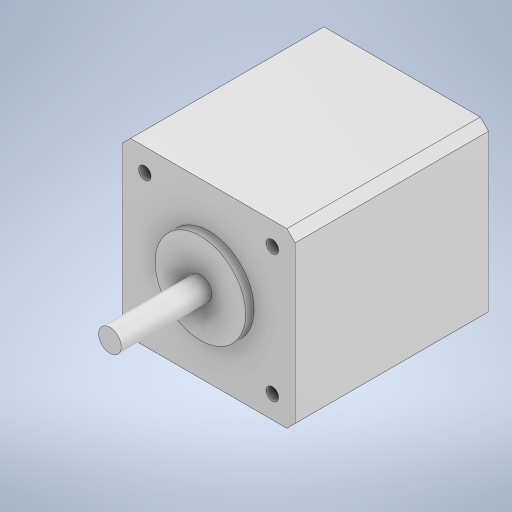
# Autodesk Inventor part: stepper motor
Saved by Autodesk Inventor 2024 (Build 280153000, 153)
## iProperties
Created: 2023-10-25
Part Number: stepper motor
Material: Aluminum
Document SubType Name: Modeling
Designer: mb
Density: 2.7 g/cm^3
Appearance: Satin
Mass: 225.957 g
Surface Area: 118.758 cm^2
Volume: 83.6877 cm^3
Author: mb
Autodesk Inventor part; units mm, degrees
ref_plane "YZ Plane" through (0, 0, 0) normal (1, 0, 0) x (0, 1, 0)
sketch "Sketch1" plane through (0, 0, 0) normal (0, 0, 1) x (1, 0, 0)
  line L0 (0, 0) -> (42, 0)
  line L1 (42, 0) -> (42, 42)
  line L2 (42, 42) -> (0, 42)
  line L3 (0, 42) -> (0, 0)
  dimension "d0" = 42
  dimension "d1" = 42
  constraints: 8 end point, 2 parallel, 1 horizontal, 1 perpendicular
  measures "d0" distance of L2.end L1.end
  measures "d1" distance of L1.end L0.end
extrude "Extrusion1" add sketch "Sketch1" along normal blind 47
chamfer "Chamfer1" distance 2 angle 45 4 edges at (42, 42, 23.5) (0, 42, 23.5) (42, 0, 23.5) (0, 0, 23.5)
sketch "Sketch2" plane through (0, 0, 47) normal (0, 0, 1) x (1, 0, 0)
  circle A0 centre (21, 21) radius 11
  line L0 (42, 2) -> (42, 40) projected
  line L1 (40, 42) -> (2, 42) projected
  point P0 (0, 0)
  point P1 (21, 42)
  dimension "d7" = 22
  dimension "d10" = 21
  dimension "d11" = 21
  constraints: 1 centre point, 1 midpoint
  measures "d7" diameter of A0
  measures "d10" distance from line of L0 A0.centre
  measures "d11" distance of point (21, 42) A0.centre
extrude "Extrusion2" add sketch "Sketch2" along normal blind 2
sketch "Sketch3" plane through (21, 21, 49) normal (0, 0, 1) x (1, 0, 0)
  circle A0 centre (0, 0) radius 2.75
  circle A1 centre (0, 0) radius 11 projected
  point P0 (-21, -21)
  dimension "d14" = 5.5
  constraints: 1 centre point, 1 concentric
  measures "d14" diameter of A0
extrude "Extrusion3" add sketch "Sketch3" along normal blind 24 from surface at -2 contours A0
sketch "Sketch4" plane through (0, 0, 47) normal (0, 0, 1) x (1, 0, 0)
  circle A0 centre (21, 21) radius 11 projected
  line L0 (2, 0) -> (0, 2) projected
  line L1 (2, 0) -> (40, 0) projected
  line L2 (42, 2) -> (40, 0) projected
  line L3 (42, 2) -> (42, 40) projected
  line L4 (40, 42) -> (42, 40) projected
  line L5 (40, 42) -> (2, 42) projected
  line L6 (0, 40) -> (2, 42) projected
  line L7 (0, 40) -> (0, 2) projected
  circle A1 centre (21, 21) radius 2.75 projected
  circle A2 centre (21, 21) radius 11 projected
  circle A3 centre (21, 21) radius 2.75 projected
  line L8 (5.5, 5.5) -> (36.5, 5.5)
  line L9 (36.5, 5.5) -> (36.5, 36.5)
  line L10 (36.5, 36.5) -> (5.5, 36.5)
  line L11 (5.5, 36.5) -> (5.5, 5.5)
  line L12 (5.5, 5.5) -> (36.5, 36.5) construction
  line L13 (36.5, 5.5) -> (5.5, 36.5) construction
  circle A4 centre (5.5, 5.5) radius 1.5
  circle A5 centre (5.5, 36.5) radius 1.5
  circle A6 centre (36.5, 36.5) radius 1.5
  circle A7 centre (36.5, 5.5) radius 1.5
  point P0 (0, 0)
  dimension "d17" = 31
  dimension "d18" = 31
  dimension "d19" = 3
  constraints: 12 end point, 4 centre point, 4 coincident, 3 equal radius, 2 midpoint, 2 parallel, 1 horizontal, 1 perpendicular
  measures "d17" distance of L9.end L10.end
  measures "d18" distance of L10.end L8.start
  measures "d19" diameter of A4
extrude "Extrusion4" cut sketch "Sketch4" against normal blind 4.5 contours L11 A4 L8 | L8 A4 L11 | A7 L9 L8 | L8 L9 A7 | A5 L10 L11 | L11 L10 A5 | A6 L10 L9 | L9 L10 A6
ref_plane "Work Plane1" through (21, 2, 0) normal (1, 0, 0) x (0, 0, -1)
ref_plane "Work Plane2" through (21, 2, 0) normal (1, 0, 0) x (0, 0, -1)
body "Solid1"
